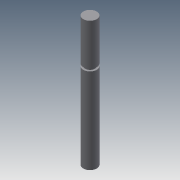
# Autodesk Inventor part: hridelka2
Saved by Autodesk Inventor 2013 (Build 170138000, 138)
## iProperties
Created: 2013-05-13
Part Number: hridelka2
Material: Generic
Document SubType Name: Modeling
Designer: idle-rug
Density: 1 g/cm^3
Author: idle-rug
Autodesk Inventor part; units mm, degrees
ref_plane "YZ Plane" through (0, 0, 0) normal (1, 0, 0) x (0, 1, 0)
ref_plane "XZ Plane" through (0, 0, 0) normal (0, 1, 0) x (-1, 0, 0)
ref_plane "XY Plane" through (0, 0, 0) normal (0, 0, 1) x (1, 0, 0)
sketch "Sketch1" plane through (0, 0, 0) normal (0, 1, 0) x (-1, 0, 0)
  point P0 (0, 0)
sketch "Sketch2" plane through (0, 0, 0) normal (1, 0, 0) x (0, 1, 0)
  line L0 (0, -29.75) -> (3, -29.75)
  line L1 (3, 8.25) -> (2.15, 8.25)
  line L2 (2.15, 8.25) -> (2.15, 9.25)
  line L3 (2.15, 9.25) -> (3, 9.25)
  line L4 (3, 9.25) -> (3, 27.75)
  line L5 (3, 8.25) -> (3, -29.75)
  line L6 (3, 27.75) -> (0, 27.75)
  line L7 (0, 27.75) -> (0, -29.75)
  line L8 (0, -41.25) -> (0, 39.25) projected
  point P0 (0, 0)
  dimension "d6" = 0.85
  dimension "d7" = 1
  constraints: 16 end point, 3 perpendicular, 1 horizontal
  measures "d6" distance of L1.start L1.end
  measures "d7" distance of L1.end L2.end
revolve "Revolution1" add sketch "Sketch2" angle 360 about axis through (0, 0, -10) along (0, 0, 1)
body "Solid1"
